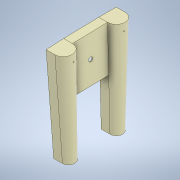
# Autodesk Inventor part: Prototip1
Saved by Autodesk Inventor 2020.3 (Build 243373000, 373)
## iProperties
Created: 2021-03-12
Part Number: Prototip1
Material: ABS Plastic
Document SubType Name: Modeling
Designer: alexo
Density: 1.06 g/cm^3
Appearance: Smooth - Ash
Author: alexo
Autodesk Inventor part; units mm, degrees
ref_plane "YZ Plane" through (0, 0, 0) normal (1, 0, 0) x (0, 1, 0)
sketch "Sketch1" plane through (0, 0, 0) normal (0, 1, 0) x (-1, 0, 0)
  line L0 (-25, -25) -> (0, -25) construction
  line L1 (25, -25) -> (25, 25)
  line L2 (25, 25) -> (0, 25)
  line L3 (-25, 25) -> (-25, -25) construction
  line L4 (-25, -25) -> (25, 25) construction
  line L5 (25, -25) -> (-25, 25) construction
  arc A0 (0, 25) -> (0, -25) centre (0, 0) ccw
  arc A1 (17.67767, 17.67767) -> (0, 25) centre (0, 0) ccw construction
  arc A2 (0, -25) -> (17.67767, 17.67767) centre (0, 0) ccw construction
  line L6 (0, 25) -> (-25, 25) construction
  line L7 (0, -25) -> (25, -25)
  point P0 (0, 0)
  dimension "d0" = 50
  dimension "d1" = 50
  dimension "d2" = 25
  constraints: 16 end point, 6 point on circle, 5 parallel, 3 centre point, 2 horizontal, 2 midpoint, 2 perpendicular, 1 coincident, 1 point on line
  measures "d0" distance between parallel lines of L7 L2
  measures "d1" distance between parallel lines of L3 L1
  measures "d2" radius of A0
ref_plane "Work Plane2" through (-25, -280, 25) normal (0, -1, 0) x (1, 0, 0)
ref_plane "Work Plane1" through (-25, 0, 25) normal (0, -1, 0) x (1, 0, 0)
sketch "Sketch2" plane through (-25, -280, 25) normal (0, -1, 0) x (1, 0, 0)
  arc A0 (25, -42.857143) -> (25, -7.142857) centre (25, -25) ccw
  line L0 (25, -42.857143) -> (0, -42.857143)
  line L1 (0, -50) -> (0, 0)
  line L2 (25, -7.142857) -> (0, -7.142857)
  arc A1 (25, -7.142857) -> (25, -42.857143) centre (25, -25) ccw construction
  dimension "d4" = 35.71429
  constraints: 4 end point, 4 point on circle, 2 centre point, 2 point on line, 2 tangent, 1 coincident, 1 horizontal, 1 perpendicular
  measures "d4" diameter of A0
sketch "Sketch1 outline for Loft1" plane through (0, 0, 0) normal (0, 1, 0) x (-1, 0, 0)
  line L0 (25, 25) -> (25, -25)
  line L1 (25, -25) -> (0, -25)
  arc A0 (0, -25) -> (0, 25) centre (0, 0) cw
  line L2 (0, 25) -> (25, 25)
sketch "Sketch2 outline for Loft1" plane through (-25, -280, 25) normal (0, -1, 0) x (1, 0, 0)
  line L0 (0, -42.857143) -> (25, -42.857143)
  line L1 (0, -7.142857) -> (0, -42.857143)
  line L2 (25, -7.142857) -> (0, -7.142857)
  arc A0 (25, -42.857143) -> (25, -7.142857) centre (25, -25) ccw
loft "Loft1" add profiles "Sketch1 outline for Loft1", "Sketch2 outline for Loft1"
shell "Shell1" thickness 2 removed faces 1 at (-25, -11.666667, 2.058532)
ref_plane "Work Plane4" through (-25, -1.275095, 74.983739) normal (0, -0.0255019, 0.9996748) x (1, 0, 0)
mirror "Mirror1" about plane through (-25, -1.275095, 74.983739) normal (0, -0.0255019, 0.9996748)
sketch "Sketch3" plane through (-25, 0, 25) normal (0, -0.0255019, 0.9996748) x (1, 0, 0)
  line L0 (25, 0) -> (0, 0)
  line L1 (0, 0) -> (0, -280.091093)
  line L2 (25, -280.091093) -> (0, -280.091093)
  line L3 (25, 0) -> (25, -280.091093)
  line L4 (25, 0) -> (0, 0)
  line L5 (0, 0) -> (0, -132)
  line L6 (0, -132) -> (25, -132)
  line L7 (25, -132) -> (25, 0)
  point P0 (25, -0.637548)
  point P1 (0, -132)
  point P2 (25, -132)
  dimension "d12" = 132
  constraints: 8 end point, 2 parallel, 1 horizontal, 1 perpendicular
  measures "d12" distance between parallel lines of L0 L6
sketch "Sketch3 outline for Extrusion1" plane through (-25, 0, 25) normal (0, -0.0255019, 0.9996748) x (1, 0, 0)
  line L0 (0, -132) -> (25, -132)
  line L1 (0, 0) -> (0, -132)
  line L2 (25, 0) -> (0, 0)
  line L3 (25, -132) -> (25, 0)
extrude "Extrusion1" add sketch "Sketch3 outline for Extrusion1" along normal up to surface (100 mm away)
shell "Shell2" thickness 2 removed faces 1 at (-25, -47.053153, 90.48802)
sketch "Sketch4" plane through (0, -134.507261, 121.601226) normal (1, 0, 0) x (0, 0.0255019, -0.9996748)
  line L0 (100, 132) -> (149.983739, 130.724905) construction
  line L1 (100, 132) -> (0, 0) construction
  circle A0 centre (50, 66) radius 6
  point P0 (124.991869, 131.362452)
  dimension "d16" = 12
  constraints: 2 end point, 1 centre point, 1 midpoint
  measures "d16" diameter of A0
sketch "Sketch4 outline for Extrusion2" plane through (0, -134.507261, 121.601226) normal (1, 0, 0) x (0, 0.0255019, -0.9996748)
  circle A0 centre (50, 66) radius 6
extrude "Extrusion2" cut sketch "Sketch4 outline for Extrusion2" against normal through all
sketch "Sketch5" plane through (-25, -280, -17.857143) normal (-1, 0, 0) x (0, 0, 1)
  circle A0 centre (164.256423, 254.895922) radius 1.5
  circle A1 centre (20.303256, 258.568197) radius 1.5
  point P0 (17.857143, 280)
sketch "Sketch5 outline for Extrusion3" plane through (-25, -280, -17.857143) normal (-1, 0, 0) x (0, 0, 1)
  circle A0 centre (164.256423, 254.895922) radius 1.5
  circle A1 centre (20.303256, 258.568197) radius 1.5
extrude "Extrusion3" cut sketch "Sketch5 outline for Extrusion3" against normal through all
equation "\"d0\" = LatimeB"
equation "\"d1\" = d0"
equation "\"d2\" = 0.5 * LatimeB"
equation "\"d12\" = Platforma"
equation "\"LatimeB\" = 50"
equation "\"k\" = 1.4"
equation "\"Platforma\" = 132"
body "Solid1"
